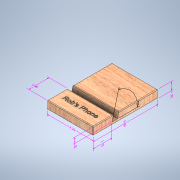
# Autodesk Inventor part: robsCopyOfMelodiesKindleStand
Saved by Autodesk Inventor 2021.1 (Build 251245000, 245)
## iProperties
Created: 2020-01-24
Part Number: robsCopyOfMelodiesKindleStand
Material: Wood (Birch)
Document SubType Name: Modeling
Designer: steele
Density: 0.55 g/cm^3
Appearance: Birch - Natural Polished
Author: steele
Autodesk Inventor part; units mm, degrees
ref_plane "YZ Plane" through (0, 0, 0) normal (1, 0, 0) x (0, 1, 0)
ref_plane "XZ Plane" through (0, 0, 0) normal (0, 1, 0) x (-1, 0, 0)
ref_plane "XY Plane" through (0, 0, 0) normal (0, 0, 1) x (1, 0, 0)
sketch "Sketch2" plane through (0, 0, 0) normal (0, 1, 0) x (-1, 0, 0)
  line L0 (53.975, 76.2) -> (-53.975, 76.2)
  line L1 (-53.975, 76.2) -> (-53.975, -76.2)
  line L2 (-53.975, -76.2) -> (53.975, -76.2)
  line L3 (53.975, -76.2) -> (53.975, 76.2)
  line L4 (53.975, 76.2) -> (-53.975, -76.2) construction
  line L5 (-53.975, 76.2) -> (53.975, -76.2) construction
  point P0 (0, 0)
  dimension "d0" = 107.95
  dimension "d1" = 152.4
  constraints: 12 end point, 2 midpoint, 2 parallel, 1 horizontal, 1 perpendicular
  measures "d0" distance of L0.start L0.end
  measures "d1" distance of L1.end L0.end
extrude "Extrusion1" add sketch "Sketch2" along normal blind 19.05
sketch "Sketch4" plane through (53.975, 0, 76.2) normal (1, 0, 0) x (0, 0, -1)
  line L0 (0, 19.05) -> (152.4, 19.05) projected
  line L1 (61.001, 19.05) -> (57.598, 6.35)
  line L2 (57.598, 6.35) -> (44.45, 6.35)
  line L3 (44.45, 6.35) -> (47.853, 19.05)
  line L4 (61.001, 19.05) -> (47.853, 19.05)
  line L5 (0, 0) -> (0, 19.05) projected
  point P0 (76.2, 0)
  point P1 (73.5162, 12.7)
  dimension "d27" = 12.7
  dimension "d28" = 44.45
  dimension "d29" = 75
  dimension "d46" = 12.7
  constraints: 8 end point, 2 parallel, 1 horizontal, 3 other
  measures "d28" distance from line of L5 L2.end
  measures "d29" angle of L3 L2
  measures "d46" distance between parallel lines of L1 L3
extrude "Extrusion3" cut sketch "Sketch4" against normal through all
sketch "Sketch6" plane through (0, 19.05, 0) normal (0, 1, 0) x (1, 0, 0)
  line L0 (-53.975, -28.347) -> (-53.975, -76.2) construction
  line L1 (-53.975, -50.8) -> (53.975, -50.8) construction
  line L2 (53.975, -76.2) -> (53.975, -28.347) construction
  line L3 (-53.975, -76.2) -> (53.975, -76.2) construction
  line L4 (-39.2964, -55.88) -> (-39.2964, -45.72)
  line L5 (-39.2964, -45.72) -> (-34.7895, -45.72)
  spline S0 degree 2 poles (-34.7895, -45.72) (-33.4343, -45.72) (-32.0172, -46.2698) (-31.1731, -47.656) (-31.1731, -48.4923) knots 0 0 0 1 2 3 3 3
  spline S1 degree 2 poles (-31.1731, -48.4923) (-31.1731, -49.5765) (-32.5747, -51.0555) (-34.0306, -51.2569) knots 0 0 0 1 2 2 2
  spline S2 degree 2 poles (-34.0306, -51.2569) (-33.504, -51.5124) (-33.2252, -51.7602) knots 0 0 0 1 1 1
  spline S3 degree 2 poles (-33.2252, -51.7602) (-32.6367, -52.3023) (-32.1101, -53.1154) knots 0 0 0 1 1 1
  line L6 (-32.1101, -53.1154) -> (-30.3522, -55.88)
  line L7 (-30.3522, -55.88) -> (-32.0327, -55.88)
  line L8 (-32.0327, -55.88) -> (-33.3801, -53.7659)
  spline S4 degree 2 poles (-33.3801, -53.7659) (-33.9686, -52.8521) (-34.7275, -51.8841) (-35.3316, -51.4892) (-35.6413, -51.4118) knots 0 0 0 1 2 3 3 3
  spline S5 degree 2 poles (-35.6413, -51.4118) (-35.8736, -51.3653) (-36.3925, -51.3653) knots 0 0 0 1 1 1
  line L9 (-36.3925, -51.3653) -> (-37.949, -51.3653)
  line L10 (-37.949, -51.3653) -> (-37.949, -55.88)
  line L11 (-37.949, -55.88) -> (-39.2964, -55.88)
  line L12 (-37.949, -50.2037) -> (-35.0605, -50.2037)
  spline S6 degree 2 poles (-35.0605, -50.2037) (-34.139, -50.2037) (-33.1013, -49.8243) (-32.5592, -48.9802) (-32.5592, -48.4923) knots 0 0 0 1 2 3 3 3
  spline S7 degree 2 poles (-32.5592, -48.4923) (-32.5592, -47.7721) (-33.6047, -46.8429) (-34.7353, -46.8429) knots 0 0 0 1 2 2 2
  line L13 (-34.7353, -46.8429) -> (-37.949, -46.8429)
  line L14 (-37.949, -46.8429) -> (-37.949, -50.2037)
  spline S8 degree 2 poles (-29.6863, -52.1939) (-29.6863, -50.1573) (-28.5479, -49.1738) knots 0 0 0 1 1 1
  spline S9 degree 2 poles (-28.5479, -49.1738) (-27.6031, -48.3529) (-26.2402, -48.3529) knots 0 0 0 1 1 1
  spline S10 degree 2 poles (-26.2402, -48.3529) (-24.7224, -48.3529) (-22.7942, -50.3431) (-22.7942, -52.0932) knots 0 0 0 1 2 2 2
  spline S11 degree 2 poles (-22.7942, -52.0932) (-22.7942, -53.5104) (-23.646, -55.1443) (-25.2722, -56.0426) (-26.2402, -56.0426) knots 0 0 0 1 2 3 3 3
  spline S12 degree 2 poles (-26.2402, -56.0426) (-27.7813, -56.0426) (-29.6863, -54.0602) (-29.6863, -52.1939) knots 0 0 0 1 2 2 2
  spline S13 degree 2 poles (-28.4008, -52.2016) (-28.4008, -53.611) (-27.1695, -55.0204) (-26.2402, -55.0204) knots 0 0 0 1 2 2 2
  spline S14 degree 2 poles (-26.2402, -55.0204) (-25.3109, -55.0204) (-24.0797, -53.6033) (-24.0797, -52.1552) knots 0 0 0 1 2 2 2
  spline S15 degree 2 poles (-24.0797, -52.1552) (-24.0797, -50.7923) (-25.3187, -49.3829) (-26.2402, -49.3829) knots 0 0 0 1 2 2 2
  spline S16 degree 2 poles (-26.2402, -49.3829) (-27.1695, -49.3829) (-28.4008, -50.7845) (-28.4008, -52.2016) knots 0 0 0 1 2 2 2
  line L15 (-20.1845, -55.88) -> (-21.3383, -55.88)
  line L16 (-21.3383, -55.88) -> (-21.3383, -45.72)
  line L17 (-21.3383, -45.72) -> (-20.0916, -45.72)
  line L18 (-20.0916, -45.72) -> (-20.0916, -49.3441)
  spline S17 degree 2 poles (-20.0916, -49.3441) (-19.3017, -48.3529) (-18.0781, -48.3529) knots 0 0 0 1 1 1
  spline S18 degree 2 poles (-18.0781, -48.3529) (-17.3967, -48.3529) (-16.1809, -48.9027) (-15.3988, -49.894) (-14.9573, -51.2879) (-14.9573, -52.0855) knots 0 0 0 1 2 3 4 4 4
  spline S19 degree 2 poles (-14.9573, -52.0855) (-14.9573, -53.975) (-16.8314, -56.0426) (-18.1401, -56.0426) knots 0 0 0 1 2 2 2
  spline S20 degree 2 poles (-18.1401, -56.0426) (-19.4411, -56.0426) (-20.1845, -54.9585) knots 0 0 0 1 1 1
  line L19 (-20.1845, -54.9585) -> (-20.1845, -55.88)
  spline S21 degree 2 poles (-20.2, -52.1397) (-20.2, -53.4639) (-19.8438, -54.0602) knots 0 0 0 1 1 1
  spline S22 degree 2 poles (-19.8438, -54.0602) (-19.2552, -55.0204) (-18.2485, -55.0204) knots 0 0 0 1 1 1
  spline S23 degree 2 poles (-18.2485, -55.0204) (-17.4354, -55.0204) (-16.2428, -53.5955) (-16.2428, -52.1939) knots 0 0 0 1 2 2 2
  spline S24 degree 2 poles (-16.2428, -52.1939) (-16.2428, -50.7458) (-17.3812, -49.3751) (-18.1943, -49.3751) knots 0 0 0 1 2 2 2
  spline S25 degree 2 poles (-18.1943, -49.3751) (-19.0074, -49.3751) (-20.2, -50.8) (-20.2, -52.1397) knots 0 0 0 1 2 2 2
  line L20 (-13.4318, -49.3209) -> (-13.7493, -47.4237)
  line L21 (-13.7493, -47.4237) -> (-13.7493, -45.72)
  line L22 (-13.7493, -45.72) -> (-12.3322, -45.72)
  line L23 (-12.3322, -45.72) -> (-12.3322, -47.4237)
  line L24 (-12.3322, -47.4237) -> (-12.6652, -49.3209)
  line L25 (-12.6652, -49.3209) -> (-13.4318, -49.3209)
  line L26 (-11.2325, -53.6807) -> (-10.0013, -53.4871)
  spline S26 degree 2 poles (-10.0013, -53.4871) (-9.9006, -54.2305) (-8.9481, -55.0204) (-8.0885, -55.0204) knots 0 0 0 1 2 2 2
  spline S27 degree 2 poles (-8.0885, -55.0204) (-7.2289, -55.0204) (-6.3926, -54.3157) (-6.3926, -53.8434) knots 0 0 0 1 2 2 2
  spline S28 degree 2 poles (-6.3926, -53.8434) (-6.3926, -53.4252) (-6.7643, -53.1774) knots 0 0 0 1 1 1
  spline S29 degree 2 poles (-6.7643, -53.1774) (-7.0198, -53.0148) (-8.042, -52.7592) knots 0 0 0 1 1 1
  spline S30 degree 2 poles (-8.042, -52.7592) (-9.4127, -52.4107) (-10.4736, -51.9074) (-11.0234, -51.0091) (-11.0234, -50.4748) knots 0 0 0 1 2 3 3 3
  spline S31 degree 2 poles (-11.0234, -50.4748) (-11.0234, -49.9791) (-10.5743, -49.1428) (-10.1871, -48.864) knots 0 0 0 1 2 2 2
  spline S32 degree 2 poles (-10.1871, -48.864) (-9.8928, -48.6472) (-8.8861, -48.3529) (-8.3053, -48.3529) knots 0 0 0 1 2 2 2
  spline S33 degree 2 poles (-8.3053, -48.3529) (-7.438, -48.3529) (-6.1293, -48.8563) (-5.502, -49.7081) (-5.3859, -50.4205) knots 0 0 0 1 2 3 3 3
  line L27 (-5.3859, -50.4205) -> (-6.6094, -50.5832)
  spline S34 degree 2 poles (-6.6094, -50.5832) (-6.6946, -50.0101) (-7.4922, -49.3751) (-8.2202, -49.3751) knots 0 0 0 1 2 2 2
  spline S35 degree 2 poles (-8.2202, -49.3751) (-9.0797, -49.3751) (-9.8154, -49.9482) (-9.8154, -50.3276) knots 0 0 0 1 2 2 2
  spline S36 degree 2 poles (-9.8154, -50.3276) (-9.8154, -50.5677) (-9.6605, -50.7613) knots 0 0 0 1 1 1
  spline S37 degree 2 poles (-9.6605, -50.7613) (-9.5134, -50.9626) (-9.1804, -51.0943) knots 0 0 0 1 1 1
  spline S38 degree 2 poles (-9.1804, -51.0943) (-8.9945, -51.164) (-8.0808, -51.4195) knots 0 0 0 1 1 1
  spline S39 degree 2 poles (-8.0808, -51.4195) (-6.7566, -51.768) (-5.7034, -52.2171) (-5.1071, -53.0767) (-5.1071, -53.7195) knots 0 0 0 1 2 3 3 3
  spline S40 degree 2 poles (-5.1071, -53.7195) (-5.1071, -54.339) (-5.835, -55.4386) (-7.2134, -56.0426) (-8.0808, -56.0426) knots 0 0 0 1 2 3 3 3
  spline S41 degree 2 poles (-8.0808, -56.0426) (-9.5134, -56.0426) (-11.0234, -54.8501) (-11.2325, -53.6807) knots 0 0 0 1 2 2 2
  line L28 (0.4685, -55.88) -> (0.4685, -45.72)
  line L29 (0.4685, -45.72) -> (4.3017, -45.72)
  spline S42 degree 2 poles (4.3017, -45.72) (5.3162, -45.72) (5.8505, -45.8207) knots 0 0 0 1 1 1
  spline S43 degree 2 poles (5.8505, -45.8207) (6.6017, -45.9446) (7.6084, -46.6415) (8.2279, -47.9038) (8.2279, -48.6627) knots 0 0 0 1 2 3 3 3
  spline S44 degree 2 poles (8.2279, -48.6627) (8.2279, -49.9559) (6.5784, -51.7525) (4.4256, -51.7525) knots 0 0 0 1 2 2 2
  line L30 (4.4256, -51.7525) -> (1.8159, -51.7525)
  line L31 (1.8159, -51.7525) -> (1.8159, -55.88)
  line L32 (1.8159, -55.88) -> (0.4685, -55.88)
  line L33 (1.8159, -50.5522) -> (4.4411, -50.5522)
  spline S45 degree 2 poles (4.4411, -50.5522) (5.7498, -50.5522) (6.8417, -49.5842) (6.8417, -48.7014) knots 0 0 0 1 2 2 2
  spline S46 degree 2 poles (6.8417, -48.7014) (6.8417, -48.0664) (6.199, -47.1526) (5.6724, -47.0132) knots 0 0 0 1 2 2 2
  spline S47 degree 2 poles (5.6724, -47.0132) (5.3317, -46.9203) (4.4179, -46.9203) knots 0 0 0 1 1 1
  line L34 (4.4179, -46.9203) -> (1.8159, -46.9203)
  line L35 (1.8159, -46.9203) -> (1.8159, -50.5522)
  line L36 (9.7844, -55.88) -> (9.7844, -45.72)
  line L37 (9.7844, -45.72) -> (11.0312, -45.72)
  line L38 (11.0312, -45.72) -> (11.0312, -49.3674)
  spline S48 degree 2 poles (11.0312, -49.3674) (11.9062, -48.3529) (13.2382, -48.3529) knots 0 0 0 1 1 1
  spline S49 degree 2 poles (13.2382, -48.3529) (14.0513, -48.3529) (15.2594, -48.9957) (15.7782, -50.134) (15.7782, -51.2182) knots 0 0 0 1 2 3 3 3
  line L39 (15.7782, -51.2182) -> (15.7782, -55.88)
  line L40 (15.7782, -55.88) -> (14.5314, -55.88)
  line L41 (14.5314, -55.88) -> (14.5314, -51.2182)
  spline S50 degree 2 poles (14.5314, -51.2182) (14.5314, -50.2812) (13.7183, -49.4293) (12.9827, -49.4293) knots 0 0 0 1 2 2 2
  spline S51 degree 2 poles (12.9827, -49.4293) (12.4251, -49.4293) (11.4494, -50.0024) (11.0312, -50.9859) (11.0312, -51.8532) knots 0 0 0 1 2 3 3 3
  line L42 (11.0312, -51.8532) -> (11.0312, -55.88)
  line L43 (11.0312, -55.88) -> (9.7844, -55.88)
  spline S52 degree 2 poles (17.2108, -52.1939) (17.2108, -50.1573) (18.3492, -49.1738) knots 0 0 0 1 1 1
  spline S53 degree 2 poles (18.3492, -49.1738) (19.2939, -48.3529) (20.6569, -48.3529) knots 0 0 0 1 1 1
  spline S54 degree 2 poles (20.6569, -48.3529) (22.1747, -48.3529) (24.1029, -50.3431) (24.1029, -52.0932) knots 0 0 0 1 2 2 2
  spline S55 degree 2 poles (24.1029, -52.0932) (24.1029, -53.5104) (23.2511, -55.1443) (21.6248, -56.0426) (20.6569, -56.0426) knots 0 0 0 1 2 3 3 3
  spline S56 degree 2 poles (20.6569, -56.0426) (19.1158, -56.0426) (17.2108, -54.0602) (17.2108, -52.1939) knots 0 0 0 1 2 2 2
  spline S57 degree 2 poles (18.4963, -52.2016) (18.4963, -53.611) (19.7276, -55.0204) (20.6569, -55.0204) knots 0 0 0 1 2 2 2
  spline S58 degree 2 poles (20.6569, -55.0204) (21.5861, -55.0204) (22.8174, -53.6033) (22.8174, -52.1552) knots 0 0 0 1 2 2 2
  spline S59 degree 2 poles (22.8174, -52.1552) (22.8174, -50.7923) (21.5784, -49.3829) (20.6569, -49.3829) knots 0 0 0 1 2 2 2
  spline S60 degree 2 poles (20.6569, -49.3829) (19.7276, -49.3829) (18.4963, -50.7845) (18.4963, -52.2016) knots 0 0 0 1 2 2 2
  line L44 (25.5665, -55.88) -> (25.5665, -48.5155)
  line L45 (25.5665, -48.5155) -> (26.6894, -48.5155)
  line L46 (26.6894, -48.5155) -> (26.6894, -49.561)
  spline S61 degree 2 poles (26.6894, -49.561) (27.5025, -48.3529) (29.028, -48.3529) knots 0 0 0 1 1 1
  spline S62 degree 2 poles (29.028, -48.3529) (29.694, -48.3529) (30.8091, -48.833) (31.3667, -49.6074) (31.4751, -50.1418) knots 0 0 0 1 2 3 3 3
  spline S63 degree 2 poles (31.4751, -50.1418) (31.5448, -50.4902) (31.5448, -51.3576) knots 0 0 0 1 1 1
  line L47 (31.5448, -51.3576) -> (31.5448, -55.88)
  line L48 (31.5448, -55.88) -> (30.298, -55.88)
  line L49 (30.298, -55.88) -> (30.298, -51.404)
  spline S64 degree 2 poles (30.298, -51.404) (30.298, -50.6451) (30.0038, -49.8862) (29.2681, -49.4371) (28.7647, -49.4371) knots 0 0 0 1 2 3 3 3
  spline S65 degree 2 poles (28.7647, -49.4371) (27.9671, -49.4371) (26.8133, -50.4515) (26.8133, -51.8609) knots 0 0 0 1 2 2 2
  line L50 (26.8133, -51.8609) -> (26.8133, -55.88)
  line L51 (26.8133, -55.88) -> (25.5665, -55.88)
  line L52 (38.4911, -53.5026) -> (39.7843, -53.6652)
  spline S66 degree 2 poles (39.7843, -53.6652) (39.4745, -54.7959) (37.8251, -56.0426) (36.5473, -56.0426) knots 0 0 0 1 2 2 2
  spline S67 degree 2 poles (36.5473, -56.0426) (34.9289, -56.0426) (33.0394, -54.0524) (33.0394, -52.2636) knots 0 0 0 1 2 2 2
  spline S68 degree 2 poles (33.0394, -52.2636) (33.0394, -50.4051) (34.9521, -48.3529) (36.4777, -48.3529) knots 0 0 0 1 2 2 2
  spline S69 degree 2 poles (36.4777, -48.3529) (37.949, -48.3529) (39.823, -50.3663) (39.823, -52.1862) knots 0 0 0 1 2 2 2
  spline S70 degree 2 poles (39.823, -52.1862) (39.823, -52.2946) (39.8153, -52.5191) knots 0 0 0 1 1 1
  line L53 (39.8153, -52.5191) -> (34.3248, -52.5191)
  spline S71 degree 2 poles (34.3248, -52.5191) (34.3945, -53.7349) (35.6258, -55.0204) (36.5473, -55.0204) knots 0 0 0 1 2 2 2
  spline S72 degree 2 poles (36.5473, -55.0204) (37.2366, -55.0204) (38.2045, -54.2925) (38.4911, -53.5026) knots 0 0 0 1 2 2 2
  line L54 (34.3945, -51.497) -> (38.5066, -51.497)
  spline S73 degree 2 poles (38.5066, -51.497) (38.4214, -50.5677) (38.0342, -50.0953) knots 0 0 0 1 1 1
  spline S74 degree 2 poles (38.0342, -50.0953) (37.4379, -49.3751) (36.4854, -49.3751) knots 0 0 0 1 1 1
  spline S75 degree 2 poles (36.4854, -49.3751) (35.6258, -49.3751) (34.4565, -50.529) (34.3945, -51.497) knots 0 0 0 1 2 2 2
  point P0 (0, 0)
  dimension "d50" = 25.4
  constraints: 2 end point, 2 horizontal, 2 point on line
  measures "d50" distance between parallel lines of L1 L3
extrude "Extrusion4" cut sketch "Sketch6" against normal blind 2.54
fillet "Fillet1" radius 1.5875 16 edges at (0, 19.05, 15.199) (0, 19.05, 28.347) (0, 19.05, 76.2) (0, 19.05, -76.2) (-53.975, 19.05, -30.5005) (53.975, 19.05, -30.5005) (53.975, 19.05, 52.2735) (-53.975, 19.05, 52.2735) (0, 0, 76.2) (-53.975, 9.525, 76.2) (53.975, 9.525, 76.2) (53.975, 0, 0) (53.975, 9.525, -76.2) (0, 0, -76.2) (-53.975, 9.525, -76.2) (-53.975, 0, 0)
body "Solid1"
